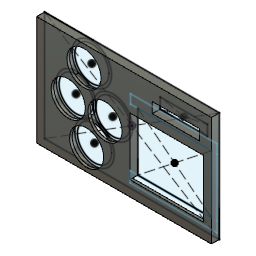
frontal_cover (Autodesk Fusion 360 design; units mm, degrees)
Autodesk Fusion 360 part; units mm, degrees
sketch "Sketch1" plane through (0, 0, 0) normal (0, 0, 1) x (1, 0, 0)
  line L0 (33.25, 20.85) -> (-33.25, 20.85)
  line L1 (-33.25, 20.85) -> (-33.25, -20.85)
  line L2 (-33.25, -20.85) -> (33.25, -20.85)
  line L3 (33.25, -20.85) -> (33.25, 20.85)
  line L4 (33.25, 20.85) -> (-33.25, -20.85) construction
  line L5 (-33.25, 20.85) -> (33.25, -20.85) construction
  circle A0 centre (-21.25, -0.15) radius 6.5
  circle A1 centre (-14.25, -12.85) radius 6.5
  circle A2 centre (-15.25, 12.85) radius 6.5
  circle A3 centre (-7.25, -0.65) radius 6.5
  line L6 (30.25, 6.85) -> (2.25, 6.85)
  line L7 (2.25, 6.85) -> (2.25, -15.15)
  line L8 (2.25, -15.15) -> (30.25, -15.15)
  line L9 (30.25, -15.15) -> (30.25, 6.85)
  line L10 (30.25, 6.85) -> (2.25, -15.15) construction
  line L11 (2.25, 6.85) -> (30.25, -15.15) construction
  line L12 (28.75, 10.85) -> (10.75, 10.85)
  line L13 (10.75, 10.85) -> (10.75, 14.85)
  line L14 (10.75, 14.85) -> (28.75, 14.85)
  line L15 (28.75, 14.85) -> (28.75, 10.85)
  line L16 (28.75, 10.85) -> (10.75, 14.85) construction
  line L17 (10.75, 10.85) -> (28.75, 14.85) construction
  point P0 (16.25, -4.15)
  point P1 (19.75, 12.85)
  dimension "d1" = 66.5
  dimension "d2" = 41.7
  dimension "d3" = 13
  dimension "d4" = 21
  dimension "d5" = 12
  dimension "d7" = 13
  dimension "d8" = 19
  dimension "d9" = 8
  dimension "d10" = 13
  dimension "d11" = 8
  dimension "d12" = 18
  dimension "d13" = 13
  dimension "d14" = 21.5
  dimension "d15" = 26
  dimension "d16" = 22
  dimension "d17" = 28
  dimension "d18" = 3
  dimension "d19" = 14
  dimension "d20" = 18
  dimension "d21" = 4
  dimension "d22" = 4.5
  dimension "d23" = 6
  constraint perpendicular L0 L1
  constraint parallel L0 L2
  constraint parallel L1 L3
  constraint horizontal L0
  constraint coincident L4 origin
  constraint coincident L5 origin
  constraint perpendicular L6 L7
  constraint parallel L6 L8
  constraint parallel L7 L9
  constraint horizontal L6
  constraint coincident L10 P0
  constraint coincident L11 P0
  constraint perpendicular L12 L13
  constraint parallel L12 L14
  constraint parallel L13 L15
  constraint horizontal L12
  constraint coincident L16 P1
  constraint coincident L17 P1
  measures "d1" distance of L1.end L2.end
  measures "d2" distance of L0.end L1.end
  measures "d3" diameter of A0
  measures "d4" distance of L0 A0.centre
  measures "d5" distance of L1 A0.centre
  measures "d7" diameter of A1
  measures "d8" distance of L1 A1.centre
  measures "d9" distance of L2 A1.centre
  measures "d10" diameter of A2
  measures "d11" distance of L0 A2.centre
  measures "d12" distance of L1 A2.centre
  measures "d13" diameter of A3
  measures "d14" distance of L0 A3.centre
  measures "d15" distance of L1 A3.centre
  measures "d16" distance of L6.end L7.end
  measures "d17" distance of L7.end L8.end
  measures "d18" distance of L3 L9
  measures "d19" distance of L0 L6
  measures "d20" distance of L13.end L14.end
  measures "d21" distance of L12.end L13.end
  measures "d22" distance of L3 L15
  measures "d23" distance of L0 L14
extrude "Extrude1" add sketch "Sketch1" along normal blind 3
sketch "Sketch3" plane through (0, 0, 0) normal (0, 0, -1) x (-1, 0, 0)
  line L0 (-28.75, 14.85) -> (-10.75, 14.85)
  line L1 (-10.75, 14.85) -> (-10.75, 10.85)
  line L2 (-10.75, 10.85) -> (-28.75, 10.85)
  line L3 (-28.75, 10.85) -> (-28.75, 14.85)
  circle A0 centre (7.25, -0.65) radius 6.5
  circle A1 centre (14.25, -12.85) radius 6.5
  circle A2 centre (15.25, 12.85) radius 6.5
  circle A3 centre (21.25, -0.15) radius 6.5
  line L4 (-30.25, -15.15) -> (-30.25, 6.85)
  line L5 (-30.25, 6.85) -> (-2.25, 6.85)
  line L6 (-2.25, 6.85) -> (-2.25, -15.15)
  line L7 (-2.25, -15.15) -> (-30.25, -15.15)
  line L8 (-33.25, 20.85) -> (-33.25, -20.85)
  line L9 (-33.25, -20.85) -> (33.25, -20.85)
  line L10 (33.25, -20.85) -> (33.25, 20.85)
  line L11 (33.25, 20.85) -> (-33.25, 20.85)
  line L12 (-30.25, -15.15) -> (0.6587, -15.15)
  line L13 (0.6587, -15.15) -> (0.6587, -19.1542)
  line L14 (0.6587, -19.1542) -> (-32.36, -19.1542)
  line L15 (-32.36, -19.1542) -> (-32.36, -15.1495)
  line L16 (-30.25, 6.8468) -> (0.5312, 6.8468)
  line L17 (0.5312, 6.8468) -> (0.5312, 10.2582)
  line L18 (0.5312, 10.2582) -> (-32.36, 10.2582)
  line L19 (-32.36, 10.2582) -> (-32.36, 6.8468)
  circle A4 centre (15.25, 12.85) radius 7.5
  circle A5 centre (21.25, -0.15) radius 7.5
  circle A6 centre (7.25, -0.65) radius 7.5
  circle A7 centre (14.25, -12.85) radius 7.5
  line L20 (-32.36, 6.8468) -> (-32.36, -15.1495)
  line L21 (-30.25, -15.15) -> (-30.25, 6.8468)
  dimension "d29" = 15
  dimension "d30" = 15
  dimension "d31" = 15
  dimension "d32" = 15
  constraint horizontal L12
  constraint vertical L13
  constraint horizontal L14
  constraint vertical L15
  constraint horizontal L16
  constraint vertical L17
  constraint horizontal L18
  constraint vertical L19
  constraint concentric A2 A4
  constraint concentric A3 A5
  constraint concentric A0 A6
  constraint concentric A1 A7
  constraint vertical L20
  constraint vertical L21
  constraint coincident L19.end L20.start
  measures "d29" diameter of A4
  measures "d30" diameter of A5
  measures "d31" diameter of A6
  measures "d32" diameter of A7
extrude "Extrude6" cut sketch "Sketch3" against normal blind 2 contours L4 L5 L6 L7 L12 L13 L14 L15 L16 L17 L18 L19 L20 L21
extrude "Extrude3" cut sketch "Sketch3" against normal blind 2 contours A4 A5 | A4 A5 A6 A7 | A5 A6 | A5 A6 A7 | A6 A7 | A5 A6 A7 picked at (10.002, 7.9892) picked at (7.8673, -7.7759) picked at (8.4052, -8.727)
